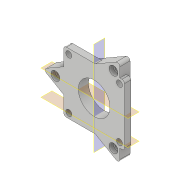
# Autodesk Inventor part: 20_Cube_Insert_Openflexure_Deltastage_Adapter
Saved by Autodesk Inventor 2019 (Build 230136000, 136)
## iProperties
Created: 2019-11-15
Part Number: 20_Cube_Insert_Openflexure_Deltastage_Adapter
Material: Generic
Document SubType Name: Modeling
Designer: diederichbenedict
Density: 1 g/cm^3
Appearance: Default
Author: diederichbenedict
Autodesk Inventor part; units mm, degrees
ref_plane "YZ Plane" through (0, 0, 0) normal (1, 0, 0) x (0, 1, 0)
ref_plane "XZ Plane" through (0, 0, 0) normal (0, 1, 0) x (-1, 0, 0)
ref_plane "XY Plane" through (0, 0, 0) normal (0, 0, 1) x (1, 0, 0)
sketch "Sketch1" plane through (0, 0, 0) normal (0, 0, 1) x (1, 0, 0)
  line L0 (15.2998, 26.5) -> (15.2998, -26.5) construction
  line L1 (15.2998, -26.5) -> (-30.5996, 0) construction
  line L2 (-30.5996, 0) -> (15.2998, 26.5) construction
  line L3 (0, 48.0119) -> (0, -48.0119) projected
  circle A0 centre (0, 0) radius 12.5
  line L4 (24.9, -24.45) -> (-24.9, -24.45) construction
  line L5 (-24.9, -24.45) -> (-24.9, 24.45) construction
  line L6 (-24.9, 24.45) -> (24.9, 24.45) construction
  line L7 (24.9, 24.45) -> (24.9, -24.45) construction
  line L8 (24.9, -24.45) -> (-24.9, 24.45) construction
  line L9 (-24.9, -24.45) -> (24.9, 24.45) construction
  line L10 (20, -20) -> (-20, -20) construction
  line L11 (-20, -20) -> (-20, 20) construction
  line L12 (-20, 20) -> (20, 20) construction
  line L13 (20, 20) -> (20, -20) construction
  line L14 (20, -20) -> (-20, 20) construction
  line L15 (-20, -20) -> (20, 20) construction
  line L16 (-37.5996, -1.7321) -> (17.2998, -33.4282)
  line L17 (20.2998, -31.6962) -> (20.2998, 31.6962)
  line L18 (17.2998, 33.4282) -> (-37.5996, 1.7321)
  arc A1 (-37.5996, 1.7321) -> (-37.5996, -1.7321) centre (-36.5996, 0) ccw
  arc A2 (20.2998, 31.6962) -> (17.2998, 33.4282) centre (18.2998, 31.6962) ccw
  arc A3 (17.2998, -33.4282) -> (20.2998, -31.6962) centre (18.2998, -31.6962) ccw
  circle A4 centre (15.2998, 26.5) radius 2
  circle A5 centre (-30.5996, 0) radius 2
  circle A6 centre (15.2998, -26.5) radius 2
  dimension "d1" = 53
  dimension "d2" = 25
  dimension "d3" = 49.8
  dimension "d4" = 48.9
  dimension "d5" = 40
  dimension "d6" = 40
  dimension "d7" = 5
  dimension "d8" = 2
  dimension "d9" = 4
  dimension "d10" = 4
  dimension "d11" = 4
  constraints: 36 end point, 7 centre point, 6 point on circle, 6 tangent, 5 coincident, 5 parallel, 4 midpoint, 2 equal radius, 2 horizontal, 2 perpendicular, 9 other
  measures "d1" distance of L0.end L0.start
  measures "d2" diameter of A0
  measures "d3" distance of L5.end L6.end
  measures "d4" distance of L4.end L5.end
  measures "d5" distance of L11.end L12.end
  measures "d6" distance of L10.end L11.end
  measures "d7" distance between parallel lines of L1 L16
  measures "d8" radius of A1
  measures "d9" diameter of A4
  measures "d10" diameter of A5
  measures "d11" diameter of A6
extrude "Extrusion1" add sketch "Sketch1" along normal blind 3 contours L18 A2 L17 A3 L16 L3 A0 | L3 A0 L16 A1 L18
sketch "Sketch3" plane through (0, 0, 3) normal (0, 0, 1) x (1, 0, 0)
  circle A0 centre (0, 0) radius 12.5 projected
  circle A1 centre (15.2998, -26.5) radius 2 projected
  circle A2 centre (-30.5996, 0) radius 2 projected
  circle A3 centre (15.2998, 26.5) radius 2 projected
  line L0 (-37.5996, -1.7321) -> (17.2998, -33.4282) projected
  arc A4 (17.2998, -33.4282) -> (20.2998, -31.6962) centre (18.2998, -31.6962) ccw projected
  line L1 (20.2998, -31.6962) -> (20.2998, 31.6962) projected
  arc A5 (20.2998, 31.6962) -> (17.2998, 33.4282) centre (18.2998, 31.6962) ccw projected
  line L2 (17.2998, 33.4282) -> (-37.5996, 1.7321) projected
  arc A6 (-37.5996, 1.7321) -> (-37.5996, -1.7321) centre (-36.5996, 0) ccw projected
  line L3 (22, -24) -> (-22, -24)
  line L4 (-24, -22) -> (-24, 22)
  line L5 (-22, 24) -> (22, 24)
  line L6 (24, 22) -> (24, -22)
  line L7 (24, -24) -> (-24, 24) construction
  line L8 (-24, -24) -> (24, 24) construction
  arc A7 (-22, 24) -> (-24, 22) centre (-22, 22) ccw
  arc A8 (-24, -22) -> (-22, -24) centre (-22, -22) ccw
  arc A9 (22, -24) -> (24, -22) centre (22, -22) ccw
  arc A10 (24, 22) -> (22, 24) centre (22, 22) ccw
  line L9 (17.2998, 33.4282) -> (-37.5996, 1.7321) projected
  line L10 (-37.5996, -1.7321) -> (17.2998, -33.4282) projected
  line L11 (20.2998, -31.6962) -> (20.2998, 31.6962) projected
  point P0 (20.2998, 24)
  point P1 (-24, 9.5838)
  point P2 (-24, -9.5838)
  point P3 (0.9697, -24)
  point P4 (20.2998, -24)
  dimension "d14" = 48
  dimension "d15" = 48
  dimension "d16" = 2
  constraints: 18 point on line, 12 end point, 8 point on circle, 8 tangent, 4 centre point, 3 equal radius, 2 midpoint, 2 parallel, 1 horizontal, 1 perpendicular
  measures "d14" distance of L7.end L8.end
  measures "d15" distance between parallel lines of L3 L5
  measures "d16" radius of A7
extrude "Extrusion2" add sketch "Sketch3" along normal blind 5 contours A0 | A1 | A3 | A6 L2 L4 L0 | L4 L2 L5 L1 L3 L0 | L0 L3 A8 L4 | L3 L1 A4 L0 | L4 A7 L5 L2 | L1 L5 A10 L6 A9 L3 | L2 A5 L1 L5
sketch "Sketch4" plane through (0, 0, 8) normal (0, 0, 1) x (1, 0, 0)
  circle A0 centre (0, 0) radius 12.5 projected
  line L0 (20, -20) -> (-20, -20) construction
  line L1 (-20, -20) -> (-20, 20) construction
  line L2 (-20, 20) -> (20, 20) construction
  line L3 (20, 20) -> (20, -20) construction
  line L4 (20, -20) -> (-20, 20) construction
  line L5 (-20, -20) -> (20, 20) construction
  circle A1 centre (15.2998, 26.5) radius 2 projected
  circle A2 centre (15.2998, -26.5) radius 2 projected
  dimension "d19" = 40
  dimension "d20" = 40
  constraints: 12 end point, 2 midpoint, 2 parallel, 1 horizontal, 1 perpendicular
  measures "d19" distance of L1.end L2.end
  measures "d20" distance of L0.end L1.end
extrude "Extrusion3" cut sketch "Sketch4" against normal through all
ref_plane "Work Plane1" through (-22, 0, 3) normal (0, 1, 0) x (1, 0, 0)
ref_plane "Work Plane2" through (0, -22, 3) normal (-1, 0, 0) x (0, 0, 1)
ref_plane "Work Plane3" through (-22, -20, 3) normal (0, 1, 0) x (1, 0, 0)
sketch "Sketch5" plane through (-22, -20, 3) normal (0, 1, 0) x (1, 0, 0)
  line L0 (22.9697, 0) -> (22.9697, -5) projected
  line L1 (22.9697, 0) -> (0, 0) projected
  line L2 (0, 0) -> (0, -5) projected
  line L3 (22.9697, -5) -> (0, -5) projected
  circle A0 centre (2, -4.2) radius 2.5
  line L4 (22, -11.7547) -> (22, 5.4591) projected
  line L5 (-0.5, -4.2) -> (4.5, -4.2)
  line L6 (0, 0) -> (0, -5) projected
  point P0 (22, 3)
  dimension "d24" = 5
  dimension "d25" = 20
  dimension "d26" = 0.8
  constraints: 2 end point, 2 point on circle, 1 centre point, 1 horizontal, 1 other
  measures "d24" diameter of A0
  measures "d25" distance from line of A0.centre L4
  measures "d26" distance from line of A0.centre L3
revolve "Revolution1" cut sketch "Sketch5" angle 360 about axis through (-22.5, -20, 7.2) along (1, 0, 0) contours A0 L5 L2 L3 | L3 L2 L5 A0
pattern_linear "Rectangular Pattern1" count 2 spacing 40 along (1, 0, 0) count 2 spacing 40 along (0, 1, 0) of "Revolution1"
sketch "Sketch6" plane through (0, 0, 8) normal (0, 0, 1) x (1, 0, 0)
  circle A0 centre (20, 20) radius 2.3685 projected
  circle A1 centre (-20, 20) radius 2.3685 projected
  circle A2 centre (20, -20) radius 2.3685 projected
  circle A3 centre (-20, -20) radius 2.3685 projected
  circle A4 centre (15.2998, -26.5) radius 2 projected
  circle A5 centre (15.2998, 26.5) radius 2 projected
  circle A6 centre (0, 0) radius 12.5 projected
  circle A7 centre (-30.5996, 0) radius 2 projected
  line L0 (0.9697, 24) -> (-22, 24) projected
  arc A8 (-22, 24) -> (-24, 22) centre (-22, 22) ccw projected
  line L1 (-24, 22) -> (-24, 9.5838) projected
  line L2 (-24, 9.5838) -> (-37.5996, 1.7321) projected
  arc A9 (-37.5996, 1.7321) -> (-37.5996, -1.7321) centre (-36.5996, 0) ccw projected
  line L3 (-37.5996, -1.7321) -> (-24, -9.5838) projected
  line L4 (-24, -9.5838) -> (-24, -22) projected
  arc A10 (-24, -22) -> (-22, -24) centre (-22, -22) ccw projected
  line L5 (-22, -24) -> (0.9697, -24) projected
  line L6 (0.9697, -24) -> (17.2998, -33.4282) projected
  arc A11 (17.2998, -33.4282) -> (20.2998, -31.6962) centre (18.2998, -31.6962) ccw projected
  line L7 (20.2998, -31.6962) -> (20.2998, -24) projected
  line L8 (20.2998, -24) -> (22, -24) projected
  arc A12 (22, -24) -> (24, -22) centre (22, -22) ccw projected
  line L9 (24, -22) -> (24, 22) projected
  arc A13 (24, 22) -> (22, 24) centre (22, 22) ccw projected
  line L10 (22, 24) -> (20.2998, 24) projected
  line L11 (20.2998, 24) -> (20.2998, 31.6962) projected
  arc A14 (20.2998, 31.6962) -> (17.2998, 33.4282) centre (18.2998, 31.6962) ccw projected
  line L12 (17.2998, 33.4282) -> (0.9697, 24) projected
hole "Hole1" at (15.2998, 26.5, 8) at (15.2998, -26.5, 8) at (-30.5996, 0, 8) direction (0, 0, -1) diameter 2.8 depth 30 tip angle 118 counterbore diameter 7 counterbore depth 3.1
body "Solid1"
